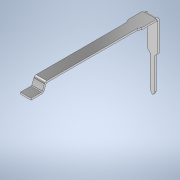
# Autodesk Inventor part: USB 3.0 A Recepticle Upper Pin
Saved by Autodesk Inventor 2020.1 (Build 241239000, 239)
## iProperties
Created: 2019-11-22
Part Number: USB 3.0 A Recepticle Upper Pin
Material: Nickel-Copper Alloy 400
Document SubType Name: Sheet Metal
Designer: S. Lee
Mass: 0.044807 g
Surface Area: 0.603272 cm^2
Volume: 0.00507441 cm^3
Density: 8.83 g/cm^3
Appearance: Chrome - Polished
Flat Pattern Width: 0.16 cm
Flat Pattern Length: 2.28127 cm
Flat Pattern Area: 0.365003 cm^2
Sheet Metal Rule: Nickel Copper Alloy
Sheet Metal Width: 1.600 mm
Sheet Metal Length: 22.813 mm
Sheet Metal Area: 36.500 mm^2
Author: S. Lee
Autodesk Inventor part; units mm, degrees
ref_plane "YZ Plane" through (0, 0, 0) normal (1, 0, 0) x (0, 1, 0)
ref_plane "XZ Plane" through (0, 0, 0) normal (0, 1, 0) x (-1, 0, 0)
ref_plane "XY Plane" through (0, 0, 0) normal (0, 0, 1) x (1, 0, 0)
sketch "Sketch1" plane through (0, 0, 0) normal (0, 1, 0) x (-1, 0, 0)
  line L0 (-0.8, 12.42) -> (0.8, 12.42)
  line L1 (0.8, 12.42) -> (0.8, 0)
  line L2 (0.8, 0) -> (-0.8, 0)
  line L3 (-0.8, 0) -> (-0.8, 12.42)
  line L4 (-0.8, 12.42) -> (0.8, 0) construction
  line L5 (0.8, 12.42) -> (-0.8, 0) construction
  line L6 (1.12, 0) -> (-1.12, 0) projected
  line L7 (0, -2.904) -> (0, 14.974) projected
  line L8 (-0.605, 0) -> (0.605, 0)
  line L9 (0.605, 0) -> (0.605, -0.35)
  line L10 (0.605, -0.35) -> (-0.605, -0.35)
  line L11 (-0.605, -0.35) -> (-0.605, 0)
  point P0 (0, 6.21)
  point P1 (-1.12, 0)
  point P2 (0, 6.21)
  dimension "d0" = 1.6
  dimension "d3" = 12.42
  dimension "d12" = 1.21
  dimension "d13" = 0.35
  constraints: 20 end point, 4 parallel, 3 horizontal, 3 midpoint, 2 perpendicular, 1 point on line, 3 other
  measures "d0" distance of L1.end L2.end
  measures "d3" distance of L0.end L1.end
  measures "d12" distance of L9.end L10.end
  measures "d13" distance of L8.end L9.end
extrude "Extrusion1" add sketch "Sketch1" along normal blind 0.2
sketch "Sketch2" plane through (0.8, 0, 12.42) normal (1, 0, 0) x (0, 0, -1)
  line L0 (0, 0.2) -> (12.42, 0.2) projected
  line L1 (-0.1349, 0.2) -> (-0.4743, -0.64)
  line L2 (-0.4743, -0.64) -> (-0.2888, -0.7149)
  line L3 (-0.2888, -0.7149) -> (0, 0)
  line L4 (0, 0) -> (12.42, 0) projected
  line L5 (-0.1349, 0.2) -> (0, 0.2)
  line L6 (0, 0) -> (0, 0.2) projected
  line L7 (0, 0.2) -> (0, 0)
  dimension "d46" = 0.2
  dimension "d47" = 112
  dimension "d48" = 112
  dimension "d49" = 0.64
  constraints: 11 end point, 1 collinear, 1 perpendicular, 1 vertical
  measures "d46" distance of L1.end L2.end
  measures "d47" angle of L4 L3
  measures "d48" angle of L5 L1
  measures "d49" distance from line of L4 L1.end
extrude "Extrusion2" add sketch "Sketch2" against normal up to surface (1.6 mm away)
sketch "Sketch3" plane through (0.8, -0.84, 14.02) normal (1, 0, 0) x (0, 0, -1)
  line L0 (14.02, 0.84) -> (1.6, 0.84) projected
  line L1 (-0.15, 0.2) -> (1.3414, 0.2)
  line L2 (1.3414, 0.2) -> (1.2606, 0)
  line L3 (1.2606, 0) -> (-0.15, 0)
  line L4 (-0.15, 0) -> (-0.15, 0.2)
  line L5 (1.3112, 0.1251) -> (1.6, 0.84) projected
  point P0 (1.1257, 0.2)
  dimension "d52" = 0.2
  dimension "d53" = 1.75
  constraints: 8 end point, 2 point on line, 1 collinear, 1 horizontal, 1 parallel, 1 perpendicular
  measures "d52" distance between parallel lines of L3 L1
  measures "d53" distance from line of L0.end L4
extrude "Extrusion3" add sketch "Sketch3" against normal up to surface (1.6 mm away)
sketch "Sketch4" plane through (0.605, 0, -0.35) normal (0, 0, -1) x (-1, 0, 0)
  line L0 (0, 0) -> (0, 0.2) projected
  line L1 (0, 0.2) -> (1.21, 0.2)
  line L2 (1.21, 0.2) -> (1.21, -3.495)
  line L3 (1.21, -3.495) -> (0, -3.495)
  line L4 (0, -3.495) -> (0, 0.2)
  line L5 (0.355, -3.495) -> (0.855, -3.495)
  line L6 (0.855, -3.495) -> (0.855, -7.81)
  line L7 (0.855, -7.81) -> (0.355, -7.81)
  line L8 (0.355, -7.81) -> (0.355, -3.495)
  line L9 (0, -3.495) -> (0.355, -3.85)
  line L10 (0, -3.495) -> (0.502, -3.495) construction
  line L11 (1.21, -3.495) -> (0.855, -3.85)
  line L12 (1.21, -3.495) -> (1.712, -3.495) construction
  line L13 (0.355, -7.477) -> (0.5184, -7.76)
  line L14 (0.6916, -7.76) -> (0.855, -7.477)
  arc A0 (0.5184, -7.76) -> (0.6916, -7.76) centre (0.605, -7.71) ccw
  line L15 (0.355, -7.477) -> (0.855, -7.477) construction
  point P0 (0.605, 0)
  dimension "d14" = 1.21
  dimension "d16" = 0.5
  dimension "d17" = 4.315
  dimension "d18" = 0.355
  dimension "d19" = 0.355
  dimension "d20" = 45
  dimension "d21" = 135
  dimension "d26" = 0.1
  dimension "d28" = 150
  dimension "d29" = 150
  dimension "d30" = 4.05
  constraints: 30 end point, 5 parallel, 5 point on line, 4 horizontal, 3 tangent, 2 equal length, 2 perpendicular, 2 point on circle, 1 centre point
  measures "d14" distance of L2.end L3.end
  measures "d16" distance of L6.end L7.end
  measures "d17" distance of L5.end L6.end
  measures "d18" distance between parallel lines of L2 L6
  measures "d19" distance between parallel lines of L4 L8
  measures "d20" angle of L9 L10
  measures "d21" angle of L11 L12
  measures "d26" radius of A0
  measures "d28" angle of L13 L8
  measures "d29" angle of L14 L6
  measures "d30" distance from line of L11.end L1
extrude "Extrusion4" add sketch "Sketch4" along normal blind 0.2 contours L0 L1 L2 L3 L4 | L3 L8 L9 | L3 L6 L14 A0 L13 L8 | L11 L6 L3
sketch "Sketch5" plane through (0, 0.2, 0) normal (0, 1, 0) x (1, 0, 0)
  line L0 (0.8, 0) -> (0.8, -12.42) projected
  line L1 (0.8, -1.6623) -> (0.605, -2)
  line L2 (-0.605, -2) -> (-0.8, -1.6623)
  line L3 (-0.8, 0) -> (-0.8, -12.5549) projected
  line L4 (0.8, -1.6623) -> (-0.8, -1.6623) construction
  line L5 (0.8, 0) -> (0.605, 0) construction
  line L6 (-0.605, 0) -> (-0.8, 0) construction
  line L7 (0.8, -1.6623) -> (0.8, -14.17)
  line L8 (-0.8, -14.17) -> (-0.8, -1.6623)
  line L9 (0.605, -2) -> (0.605, -14.17)
  line L10 (-0.605, -14.17) -> (-0.605, -2)
  line L11 (0.8, -14.17) -> (0.605, -14.17)
  line L12 (0, 3.504) -> (0, -17.174) projected
  line L13 (0.8, -14.17) -> (-0.8, -14.17) projected
  line L14 (-0.605, -14.17) -> (-0.8, -14.17)
  line L15 (-0.8, -12.8943) -> (-0.8, -14.17) projected
  point P0 (0, 0)
  point P1 (0.8, -12.62)
  point P2 (-0.8, -12.82)
  point P3 (-0.8, -12.62)
  dimension "d35" = 1.21
  dimension "d38" = 30
  dimension "d39" = 30
  dimension "d40" = 2
  constraints: 18 end point, 3 perpendicular, 3 point on line, 2 collinear, 2 parallel, 1 other
  measures "d35" distance between parallel lines of L9 L10
  measures "d38" angle of L7 L1
  measures "d39" angle of L2 L3
  measures "d40" vertical distance of L3.start L2.start
extrude "Extrusion5" cut sketch "Sketch5" against normal up to surface (1.04 mm away)
fillet "Fillet1" radius 0.3 1 edges at (0, 0, -0.35)
fillet "Fillet1" radius 0.5 1 edges at (0, 0.2, -0.55)
fillet "Fillet2" radius 0.3 2 edges at (0, 0.2, 12.5549) (0, -0.84, 12.7594)
fillet "Fillet2" radius 0.1 2 edges at (0, 0, 12.42) (0, -0.64, 12.8943)
equation "\"d48\" = d47"
equation "\"d18\" = d19"
equation "\"d39\" = d38"
equation "\"BendReliefWidth\" = Thickness"
equation "\"BendReliefDepth\" = 0.5 * Thickness"
equation "\"CornerReliefSize\" = 4 * Thickness"
equation "\"MinimumRemnant\" = 2 * Thickness"
equation "\"TransitionRadius\" = BendRadius"
equation "\"JacobiRadiusSize\" = BendRadius"
equation "\"GapSize\" = Thickness"
equation "\"Thickness\" = 0.2"
equation "\"BendRadius\" = 0.01"
body "Solid1"
